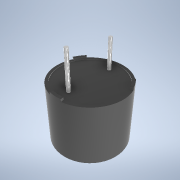
# Autodesk Inventor part: Buzzer 5v
Saved by Autodesk Inventor 2022 (Build 260153000, 153)
## iProperties
Created: 2022-06-29
Part Number: Buzzer 5v
Material: Plástico PBT
Document SubType Name: Modeling
Designer: pedro
Density: 1.31 g/cm^3
Appearance: Suave - Preto
Author: pedro
Autodesk Inventor part; units mm, degrees
ref_plane "YZ Plane" through (0, 0, 0) normal (1, 0, 0) x (0, 1, 0)
ref_plane "XZ Plane" through (0, 0, 0) normal (0, 1, 0) x (-1, 0, 0)
ref_plane "XY Plane" through (0, 0, 0) normal (0, 0, 1) x (1, 0, 0)
sketch "Esboço1" plane through (0, 0, 0) normal (0, 1, 0) x (-1, 0, 0)
  circle A0 centre (0, 0) radius 6
  dimension "d0" = 12
  constraints: 1 centre point, 1 coincident
  measures "d0" diameter of A0
extrude "Extrusão1" add sketch "Esboço1" along normal blind 9.5
sketch "Esboço2" plane through (0, 9.5, 0) normal (0, 1, 0) x (1, 0, 0)
  line L0 (0, 0) -> (0, 3.8)
  circle A0 centre (0, 3.8) radius 0.3
  dimension "d3" = 3.8
  dimension "d4" = 0.6
  constraints: 2 end point, 1 centre point, 1 coincident, 1 vertical
  measures "d3" distance of L0.start L0.end
  measures "d4" diameter of A0
extrude "Extrusão2" add sketch "Esboço2" along normal blind 5
sketch "Esboço3" plane through (0, 9.5, 0) normal (0, 1, 0) x (1, 0, 0)
  circle A0 centre (0, 3.8) radius 0.3 projected
  line L0 (0, 3.8) -> (0, -3.8)
  circle A1 centre (0, -3.8) radius 0.3
  point P0 (0, 0)
  dimension "d7" = 7.6
  constraints: 2 end point, 1 centre point, 1 coincident, 1 vertical
  measures "d7" distance of L0.start L0.end
extrude "Extrusão3" add sketch "Esboço3" along normal blind 6.2 contours A1
sketch "Esboço4" plane through (0, 9.5, 0) normal (0, 1, 0) x (1, 0, 0)
  line L0 (-0.9551, -5.4164) -> (-1.0419, -5.9088)
  circle A0 centre (0, 0) radius 6 projected
  line L1 (0, 0) -> (6, 0) construction
  line L2 (0.9551, -5.4164) -> (1.0419, -5.9088)
  arc A1 (-1.0419, -5.9088) -> (1.0419, -5.9088) centre (0, 0) ccw
  line L3 (0, -6) -> (0, -5.5)
  line L4 (1.0419, -5.9088) -> (0.9551, -5.4164)
  line L5 (-1.0419, -5.9088) -> (-0.9551, -5.4164)
  arc A2 (-0.9551, -5.4164) -> (0.9551, -5.4164) centre (0, 0) ccw
  line L6 (5.1683, 1.8811) -> (5.6382, 2.0521)
  line L7 (4.2132, 3.5353) -> (4.5963, 3.8567)
  arc A3 (5.6382, 2.0521) -> (4.5963, 3.8567) centre (0, 0) ccw
  line L8 (5.1962, 3) -> (4.7631, 2.75)
  line L9 (4.5963, 3.8567) -> (4.2132, 3.5353)
  line L10 (5.6382, 2.0521) -> (5.1683, 1.8811)
  arc A4 (5.1683, 1.8811) -> (4.2132, 3.5353) centre (0, 0) ccw
  line L11 (-4.2132, 3.5353) -> (-4.5963, 3.8567)
  line L12 (-5.1683, 1.8811) -> (-5.6382, 2.0521)
  arc A5 (-4.5963, 3.8567) -> (-5.6382, 2.0521) centre (0, 0) ccw
  line L13 (-5.1962, 3) -> (-4.7631, 2.75)
  line L14 (-5.6382, 2.0521) -> (-5.1683, 1.8811)
  line L15 (-4.5963, 3.8567) -> (-4.2132, 3.5353)
  arc A6 (-4.2132, 3.5353) -> (-5.1683, 1.8811) centre (0, 0) ccw
  dimension "d10" = 100
  dimension "d11" = 0.5
  dimension "d12" = 0.5
  dimension "d13" = 0.5
  dimension "d16" = 360
  constraints: 32 end point, 18 point on circle, 6 centre point, 1 concentric, 1 horizontal, 1 vertical, 46 other
  measures "d10" angle of L0 L1
  measures "d11" distance of L3.start L3.end
  measures "d12" distance of L2.start L2.end
  measures "d13" distance of L0.start L0.end
extrude "Extrusão4" add sketch "Esboço4" along normal blind 0.5 contours A2 L3 A0 L0 | A2 L2 A0 L3 | A0 L13 A6 L12 | A0 L11 A6 L13 | A0 L8 A4 L7 | L6 A4 L8 A0
sketch "Esboço5" plane through (0, 0, 0) normal (0, -1, 0) x (1, 0, 0)
  circle A0 centre (0, 0) radius 1.1
  dimension "d20" = 2.2
  constraints: 1 centre point, 1 coincident
  measures "d20" diameter of A0
extrude "Extrusão5" cut sketch "Esboço5" against normal blind 2
sketch "Esboço6" plane through (0, 0, 0) normal (0, -1, 0) x (1, 0, 0)
  circle A0 centre (0, 0) radius 6 projected
  line L0 (0, 6) -> (0, 4.5)
  circle A1 centre (0, 4.5) radius 1
  circle A2 centre (0, 4.5) radius 0.75
  line L1 (0, 5.25) -> (0, 5.15)
  line L2 (0, 5.15) -> (-0.2, 5.15)
  line L3 (-0.2, 5.15) -> (-0.2, 4.7)
  line L4 (-0.2, 4.7) -> (-0.65, 4.7)
  line L5 (-0.65, 4.7) -> (-0.65, 4.3)
  line L6 (-0.65, 4.3) -> (-0.2, 4.3)
  line L7 (-0.2, 4.3) -> (-0.2, 3.85)
  line L8 (-0.2, 3.85) -> (0.2, 3.85)
  line L9 (0.2, 3.85) -> (0.2, 4.3)
  line L10 (0.2, 4.3) -> (0.65, 4.3)
  line L11 (0.65, 4.3) -> (0.65, 4.7)
  line L12 (0.65, 4.7) -> (0.2, 4.7)
  line L13 (0, 5.15) -> (0.2, 5.15)
  line L14 (0.2, 5.15) -> (0.2, 4.7)
  dimension "d25" = 1.5
  dimension "d23" = 1.5
  dimension "d24" = 2
  dimension "d26" = 0.1
  dimension "d27" = 0.2
  dimension "d28" = 0.45
  dimension "d29" = 0.45
  dimension "d30" = 0.4
  dimension "d31" = 0.45
  dimension "d32" = 0.4
  dimension "d33" = 0.45
  dimension "d34" = 0.2
  constraints: 30 end point, 9 point on line, 8 perpendicular, 2 coincident, 2 vertical alignment, 1 centre point, 1 midpoint, 1 vertical, 3 other
  measures "d23" distance of L0.start L0.end
  measures "d24" diameter of A1
  measures "d26" distance of L1.start L1.end
  measures "d27" distance of L1.end L2.end
  measures "d28" distance of L2.end L3.end
  measures "d29" distance of L3.end L4.end
  measures "d30" distance of L4.end L5.end
  measures "d31" distance of L6.end L7.end
  measures "d32" distance of L7.end L8.end
  measures "d33" distance of L9.end L10.end
  measures "d34" distance of L1.end L13.end
extrude "Extrusão6" cut sketch "Esboço6" against normal blind 0.01 contours L13 L14 L12 L11 L10 L9 L8 L7 L6 L5 L4 L3 L2 | A1
sketch "Esboço7" plane through (0, 9.5, 0) normal (0, 1, 0) x (1, 0, 0)
  circle A0 centre (0, 0) radius 1.1 projected
  circle A1 centre (0, 0) radius 6
  circle A2 centre (0, 0) radius 5.5
  constraints: 2 centre point, 2 coincident
extrude "Extrusão7" add sketch "Esboço7" along normal blind 0.1 contours A1
